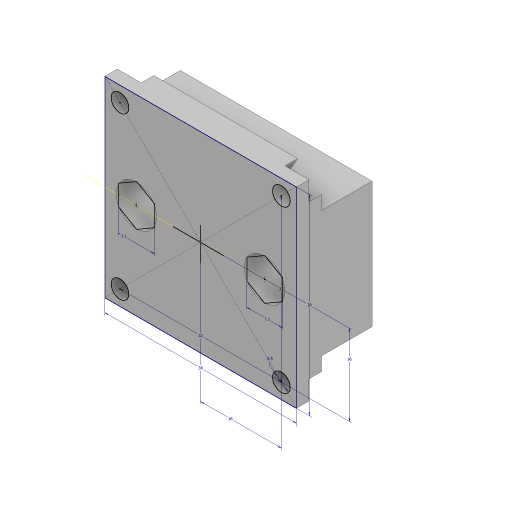
# Autodesk Inventor part: RD-PDT-S-to-M4-bolts
Saved by Autodesk Inventor 2023 (Build 270158000, 158)
## iProperties
Created: 2021-10-11
Part Number: RD-PDT-S-to-M4-bolts
Material: Generic
Document SubType Name: Modeling
Designer: Nikita
Density: 1 g/cm^3
Appearance: Default
Author: Nikita
Autodesk Inventor part; units mm, degrees
ref_plane "YZ Plane" through (0, 0, 0) normal (1, 0, 0) x (0, 1, 0)
ref_plane "XZ Plane" through (0, 0, 0) normal (0, 1, 0) x (-1, 0, 0)
ref_plane "XY Plane" through (0, 0, 0) normal (0, 0, 1) x (1, 0, 0)
sketch "Sketch5" plane through (0, 0, 0) normal (0, 0, 1) x (1, 0, 0)
  circle A0 centre (-16, 16) radius 1.75
  line L0 (-3.5516, 0) -> (2.966, 0)
  line L1 (0, 4.5757) -> (0, -5.4514)
  circle A1 centre (16, 16) radius 1.75
  circle A2 centre (-16, -16) radius 1.75
  circle A3 centre (16, -16) radius 1.75
  line L2 (19, -19) -> (-19, -19)
  line L3 (-19, -19) -> (-19, 19)
  line L4 (-19, 19) -> (19, 19)
  line L5 (19, 19) -> (19, -19)
  line L6 (19, -19) -> (-19, 19) construction
  line L7 (-19, -19) -> (19, 19) construction
  line L8 (4.0992, -12.7) -> (2.0496, -16.25)
  line L9 (2.0496, -16.25) -> (-2.0496, -16.25)
  line L10 (-2.0496, -16.25) -> (-4.0992, -12.7)
  line L11 (-4.0992, -12.7) -> (-2.0496, -9.15)
  line L12 (-2.0496, -9.15) -> (2.0496, -9.15)
  line L13 (2.0496, -9.15) -> (4.0992, -12.7)
  line L14 (4.0992, 12.7) -> (2.0496, 9.15)
  line L15 (2.0496, 9.15) -> (-2.0496, 9.15)
  line L16 (-2.0496, 9.15) -> (-4.0992, 12.7)
  line L17 (-4.0992, 12.7) -> (-2.0496, 16.25)
  line L18 (-2.0496, 16.25) -> (2.0496, 16.25)
  line L19 (2.0496, 16.25) -> (4.0992, 12.7)
  point P0 (0, 0)
  point P1 (0, 12.7)
  point P2 (0, -12.7)
  point P3 (0, -12.7)
  point P4 (0, 12.7)
  point P5 (0, -16.25)
  dimension "d47" = 3.5
  dimension "d50" = 32
  dimension "d53" = 32
  dimension "d56" = 16
  dimension "d57" = 16
  dimension "d58" = 38
  dimension "d59" = 38
  dimension "d73" = 7.1
  dimension "d74" = 7.1
  constraints: 40 end point, 4 centre point, 3 horizontal, 3 midpoint, 2 coincident, 2 parallel, 2 vertical, 1 perpendicular, 32 other
  measures "d47" diameter of A0
  measures "d50" distance of A0.centre A1.centre
  measures "d53" distance of A0.centre A2.centre
  measures "d56" distance from line of L1 A0.centre
  measures "d57" distance from line of L0 A0.centre
  measures "d58" distance of L3.end L4.end
  measures "d59" distance of L2.end L3.end
  measures "d73" distance from line of point (0, -16.25) L12
  measures "d74" distance between parallel lines of L18 L15
extrude "Extrusion3" add sketch "Sketch5" along normal blind 5 contours L2 L3 L4 L5 | L8 L9 L10 L11 L12 L13 | L14 L15 L16 L17 L18 L19
sketch "Sketch6" plane through (0, 0, 5) normal (0, 0, 1) x (1, 0, 0)
  circle A0 centre (-16, 16) radius 1.75 projected
  line L0 (-16, 19.4641) -> (-13, 17.7321)
  line L1 (-13, 17.7321) -> (-13, 14.2679)
  line L2 (-13, 14.2679) -> (-16, 12.5359)
  line L3 (-16, 12.5359) -> (-19, 14.2679)
  line L4 (-19, 14.2679) -> (-19, 17.7321)
  line L5 (-19, 17.7321) -> (-16, 19.4641)
  line L6 (0, 4.5757) -> (0, -5.4514) projected
  line L7 (-3.5516, 0) -> (2.966, 0) projected
  line L8 (16, 19.4641) -> (19, 17.7321)
  line L9 (19, 17.7321) -> (19, 14.2679)
  line L10 (19, 14.2679) -> (16, 12.5359)
  line L11 (16, 12.5359) -> (13, 14.2679)
  line L12 (13, 14.2679) -> (13, 17.7321)
  line L13 (13, 17.7321) -> (16, 19.4641)
  line L14 (-16, -12.5359) -> (-13, -14.2679)
  line L15 (-13, -14.2679) -> (-13, -17.7321)
  line L16 (-13, -17.7321) -> (-16, -19.4641)
  line L17 (-16, -19.4641) -> (-19, -17.7321)
  line L18 (-19, -17.7321) -> (-19, -14.2679)
  line L19 (-19, -14.2679) -> (-16, -12.5359)
  line L20 (16, -12.5359) -> (19, -14.2679)
  line L21 (19, -14.2679) -> (19, -17.7321)
  line L22 (19, -17.7321) -> (16, -19.4641)
  line L23 (16, -19.4641) -> (13, -17.7321)
  line L24 (13, -17.7321) -> (13, -14.2679)
  line L25 (13, -14.2679) -> (16, -12.5359)
  point P0 (0, 0)
  point P1 (-13, 16)
  point P2 (16, 16)
  point P3 (16, 16)
  point P4 (19, 16)
  point P5 (-16, -16)
  point P6 (-16, -16)
  point P7 (-13, -16)
  point P8 (16, -16)
  point P9 (16, -16)
  point P10 (19, -16)
  dimension "d62" = 6
  dimension "d65" = 32
  dimension "d68" = 32
  constraints: 48 end point, 4 coincident, 1 horizontal, 1 midpoint, 1 vertical, 58 other
  measures "d62" distance from line of point (-13, 16) L4
  measures "d65" distance of A0.centre point (16, 16)
  measures "d68" distance of A0.centre point (-16, -16)
extrude "Extrusion4" cut sketch "Sketch6" against normal blind 2.5
hole "Hole4" at (0, 12.7, 0) at (0, -12.7, 0) direction (0, 0, 1) diameter 4.2 end through all
sketch "Sketch7" plane through (0, 0, 5) normal (0, 0, 1) x (1, 0, 0)
  line L0 (-16.8038, -19) -> (-19, -17.7321) projected
  line L1 (-19, -19) -> (-19, 19) projected
  line L2 (19, -19) -> (-19, -19) projected
  line L3 (19, -19) -> (-19, 19) construction
  line L4 (-19, 17.7321) -> (-16.8038, 19) projected
  line L5 (-19, 19) -> (19, 19) projected
  line L6 (16.8038, 19) -> (19, 17.7321) projected
  line L7 (19, 19) -> (19, -19) projected
  line L8 (19, -17.7321) -> (16.8038, -19) projected
  point P0 (0, 0)
extrude "Extrusion6" cut sketch "Sketch7" against normal up to surface (2.5 mm away) contours L2 L1 L0 | L8 L7 L2 | L1 L5 L4 | L6 L5 L7
sketch "Sketch8" plane through (0, 0, 5) normal (0, 0, 1) x (1, 0, 0)
  line L0 (15.1962, 19) -> (-15.1962, 19) projected
  line L1 (12.5, -19) -> (-12.5, -19)
  line L2 (-12.5, -19) -> (-12.5, 19)
  line L3 (-12.5, 19) -> (12.5, 19)
  line L4 (12.5, 19) -> (12.5, -19)
  line L5 (12.5, -19) -> (-12.5, 19) construction
  line L6 (-12.5, -19) -> (12.5, 19) construction
  circle A0 centre (0, 12.7) radius 2.1 projected
  circle A1 centre (0, -12.7) radius 2.1 projected
  point P0 (0, 0)
  dimension "d86" = 25
  constraints: 12 end point, 2 midpoint, 2 parallel, 1 horizontal, 1 perpendicular, 1 point on line
  measures "d86" distance of L2.end L3.end
extrude "Extrusion7" add sketch "Sketch8" along normal blind 10
hole "Hole5" at (0, -12.7, 0) at (0, 12.7, 0) direction (0, 0, 1) diameter 8 depth 8
body "Solid2"
